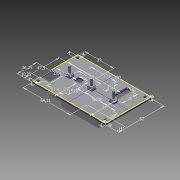
# Autodesk Inventor part: PCB-Model
Saved by Autodesk Inventor 2013 (Build 170138000, 138)
## iProperties
Created: 2013-01-14
Part Number: PCB-Model
Material: Generic
Document SubType Name: Modeling
Designer: md
Density: 1 g/cm^3
Platine_Breite: 100,000 mm
Platine_Hoehe: 62,000 mm
d26: 6,000 mm
d28: 6,000 mm
d29: 3,000 mm
Platine_Dicke: 2,000 mm
Author: md
Autodesk Inventor part; units mm, degrees
ref_plane "YZ Plane" through (0, 0, 0) normal (1, 0, 0) x (0, 1, 0)
ref_plane "XZ Plane" through (0, 0, 0) normal (0, 1, 0) x (-1, 0, 0)
ref_plane "XY Plane" through (0, 0, 0) normal (0, 0, 1) x (1, 0, 0)
sketch "Pushbutton" plane through (0, 0, 0) normal (0, 0, 1) x (1, 0, 0)
  line L0 (-3, -3) -> (3, -3)
  line L1 (3, -3) -> (3, 3)
  line L2 (3, 3) -> (-3, 3)
  line L3 (-3, 3) -> (-3, -3)
  line L4 (-3, -3) -> (3, 3) construction
  line L5 (3, -3) -> (-3, 3) construction
  circle A0 centre (0, 0) radius 1.5
  dimension "d26" = 6
  dimension "d28" = 6
  dimension "d29" = 3
  measures "d26" distance of L1.end L2.end
  measures "d28" distance of L0.end L1.end
  measures "d29" diameter of A0
sketch "Grundriss Platine" plane through (0, 0, 0) normal (0, 0, 1) x (1, 0, 0)
  line L0 (50, -31) -> (-50, -31)
  line L1 (-50, -31) -> (-50, 31)
  line L2 (-50, 31) -> (50, 31)
  line L3 (50, 31) -> (50, -31)
  line L4 (50, -31) -> (-50, 31) construction
  line L5 (-50, -31) -> (50, 31) construction
  line L6 (46, -28.52) -> (-46, -28.52) construction
  line L7 (46, -28.52) -> (-46, 28.52) construction
  line L8 (-46, -28.52) -> (46, 28.52) construction
  circle A0 centre (-46, -27) radius 2
  circle A1 centre (46, -27) radius 2
  circle A2 centre (-46, 27) radius 2
  circle A3 centre (46, 27) radius 2
  line L9 (-50, -20.75) -> (-36.6, -20.75)
  line L10 (-36.6, -20.75) -> (-36.6, -4.75)
  line L11 (-36.6, -4.75) -> (-50, -4.75)
  line L12 (-50, -4.75) -> (-50, -20.75)
  line L13 (-23, 6) -> (-15, 6)
  line L14 (-15, 6) -> (-15, -2)
  line L15 (-15, -2) -> (-23, -2)
  line L16 (-23, -2) -> (-23, 6)
  line L17 (30, 6) -> (22, 6)
  line L18 (22, 6) -> (22, 26)
  line L19 (22, 26) -> (30, 26)
  line L20 (30, 26) -> (30, 6)
  point P0 (0, 0)
  dimension "Platine_Breite" = 100
  dimension "Platine_Hoehe" = 62
  dimension "d4" = 4
  dimension "d5" = 4
  dimension "d6" = 4
  dimension "d7" = 4
  dimension "d8" = 4
  dimension "d9" = 4
  dimension "d10" = 4
  dimension "d11" = 4
  dimension "d12" = 4
  dimension "d13" = 10.25
  dimension "d14" = 13.4
  dimension "d15" = 26.25
  dimension "d16" = 29
  dimension "d17" = 27
  dimension "d18" = 8
  dimension "d19" = 8
  dimension "d20" = 37
  dimension "d21" = 8
  dimension "d22" = 72
  dimension "d23" = 20
  constraints: 42 end point, 8 parallel, 5 horizontal, 4 centre point, 4 midpoint, 4 perpendicular, 3 equal radius, 2 point on line
  measures "Platine_Breite" distance of L1.end L2.end
  measures "Platine_Hoehe" distance of L2.end L0.start
  measures "d4" diameter of A0
  measures "d5" distance from line of L0 A0.centre
  measures "d6" distance from line of A0.centre L1
  measures "d7" distance from line of A2.centre L2
  measures "d8" distance from line of A2.centre L1
  measures "d9" distance from line of A1.centre L3
  measures "d10" distance from line of A1.centre L0
  measures "d11" distance from line of A3.centre L3
  measures "d12" distance from line of A3.centre L2
  measures "d13" distance between parallel lines of L0 L9
  measures "d14" distance of L9.start L9.end
  measures "d15" distance between parallel lines of L0 L11
  measures "d16" distance between parallel lines of L0 L15
  measures "d17" distance between parallel lines of L1 L16
  measures "d18" distance of L13.start L13.end
  measures "d19" distance of L13.end L14.end
  measures "d20" distance between parallel lines of L0 L17
  measures "d21" distance of L18.end L19.end
  measures "d22" distance between parallel lines of L1 L18
  measures "d23" distance of L19.end L17.start
extrude "Extrusion1" add sketch "Grundriss Platine" along normal blind 2 contours L0 L1 L9 L10 L11 L2 L3
sketch "Bauteile Oberseite" plane through (0, 0, 2) normal (0, 0, 1) x (1, 0, 0)
  line L0 (-50, -31) -> (50, -31) projected
  line L1 (50, -31) -> (50, 31) projected
  line L2 (50, 31) -> (-50, 31) projected
  line L3 (-50, 31) -> (-50, -4.75) projected
  line L4 (-23, 6) -> (-15, 6) projected
  line L5 (-50, 0) -> (50, 0) construction
  line L6 (0, 31) -> (0, -31) construction
  line L7 (-3, -3) -> (3, -3)
  line L8 (3, -3) -> (3, 3)
  line L9 (3, 3) -> (-3, 3)
  line L10 (-3, 3) -> (-3, -3)
  line L11 (-3, -3) -> (3, 3) construction
  line L12 (3, -3) -> (-3, 3) construction
  circle A0 centre (0, 0) radius 1.5
  line L13 (-33, -3) -> (-27, -3)
  line L14 (-27, -3) -> (-27, 3)
  line L15 (-27, 3) -> (-33, 3)
  line L16 (-33, 3) -> (-33, -3)
  line L17 (-33, -3) -> (-27, 3) construction
  line L18 (-27, -3) -> (-33, 3) construction
  circle A1 centre (-30, 0) radius 1.5
  line L19 (27, -3) -> (33, -3)
  line L20 (33, -3) -> (33, 3)
  line L21 (33, 3) -> (27, 3)
  line L22 (27, 3) -> (27, -3)
  line L23 (27, -3) -> (33, 3) construction
  line L24 (33, -3) -> (27, 3) construction
  circle A2 centre (30, 0) radius 1.5
  point P0 (-30, 0)
  point P1 (0, 0)
  point P2 (30, 0)
  dimension "d30" = 30
  dimension "d31" = 30
  constraints: 4 end point, 4 midpoint, 3 point on line, 1 parallel, 6 other
extrude "Extrusion2" add sketch "Bauteile Oberseite" along normal blind 4
extrude "Extrusion3" add sketch "Bauteile Oberseite" along normal blind 12.5 contours A0 | A1 | A2
sketch "Bauteile Unterseite" plane through (0, 0, 0) normal (0, 0, -1) x (-1, 0, 0)
  line L0 (50, -20.75) -> (36.6, -20.75) projected
  line L1 (36.6, -20.75) -> (36.6, -4.75) projected
  line L2 (50, 31) -> (50, -4.75) projected
  line L3 (50, -31) -> (-50, -31) projected
  line L4 (50, -20.75) -> (50, -31) projected
  line L5 (36.6, -20.75) -> (15.2, -20.75)
  line L6 (15.2, -20.75) -> (15.2, -4.87)
  line L7 (15.2, -4.87) -> (36.6, -4.87)
  line L8 (36.6, -4.87) -> (36.6, -20.75)
  line L9 (-39.51, -30) -> (11.29, -30)
  line L10 (11.29, -30) -> (11.29, -10)
  line L11 (11.29, -10) -> (-39.51, -10)
  line L12 (-39.51, -10) -> (-39.51, -30)
  line L13 (-39.51, -30) -> (11.29, -10) construction
  line L14 (11.29, -30) -> (-39.51, -10) construction
  line L15 (27.8, 24.05) -> (-5.8, 24.05)
  line L16 (-5.8, 24.05) -> (-5.8, 8.95)
  line L17 (-5.8, 8.95) -> (27.8, 8.95)
  line L18 (27.8, 8.95) -> (27.8, 24.05)
  line L19 (27.8, 24.05) -> (-5.8, 8.95) construction
  line L20 (-5.8, 24.05) -> (27.8, 8.95) construction
  point P0 (0, 0)
  point P1 (-14.11, -20)
  point P2 (11, 16.5)
  dimension "d37" = 15.88
  dimension "d39" = 21.4
  dimension "d40" = 64.11
  dimension "d41" = 11
  dimension "d42" = 20
  dimension "d43" = 50.8
  dimension "d44" = 39
  dimension "d45" = 47.5
  dimension "d46" = 15.1
  dimension "d47" = 33.6
  constraints: 32 end point, 6 parallel, 4 midpoint, 3 horizontal, 3 perpendicular, 2 collinear
  measures "d37" distance of L5.end L6.end
  measures "d39" distance of L5.start L5.end
  measures "d40" distance from line of L4 point (-14.11, -20)
  measures "d41" distance from line of L3 point (-14.11, -20)
  measures "d42" distance of L11.end L9.start
  measures "d43" distance of L10.end L11.end
  measures "d44" distance from line of L2 point (11, 16.5)
  measures "d45" distance from line of L3 point (11, 16.5)
  measures "d46" distance of L15.end L16.end
  measures "d47" distance of L15.start L15.end
extrude "Extrusion4" add sketch "Bauteile Unterseite" along normal blind 7.7 contours L18 L17 L16 L15
extrude "Extrusion5" add sketch "Bauteile Unterseite" along normal blind 13.5 contours L5 L6 L7 L1
extrude "Extrusion6" add sketch "Bauteile Unterseite" along normal blind 10 contours L12 L11 L10 L9
equation "\"d24\" = Platine_Dicke"
equation "\"d31\" = d30"
equation "\"Platine_Dicke\" = 2"
equation "\"epsilon\" = 0.1"
equation "\"Wandstaerke\" = 3"
equation "\"Freimass\" = 3"
body "Solid1"
